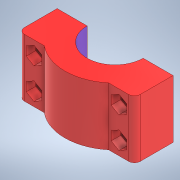
# Autodesk Inventor part: 3_Connettore_inf_INF
Saved by Autodesk Inventor 2020.2 (Build 242310000, 310)
## iProperties
Created: 2019-10-11
Part Number: 3_Connettore_inf_INF
Material: PLA(Stampato)(D0,646)
Document SubType Name: Modeling
Designer: socci
Density: 0.646 g/cm^3
Appearance: Rosso chiaro
Mass: 17.9754 g
Surface Area: 86.3527 cm^2
Volume: 27.8257 cm^3
Author: socci
Autodesk Inventor part; units mm, degrees
ref_plane "YZ Plane" through (0, 0, 0) normal (1, 0, 0) x (0, 1, 0)
ref_plane "XZ Plane" through (0, 0, 0) normal (0, 1, 0) x (-1, 0, 0)
ref_plane "XY Plane" through (0, 0, 0) normal (0, 0, 1) x (1, 0, 0)
sketch "Schizzo1" plane through (0, 0, 0) normal (0, 0, 1) x (1, 0, 0)
  line L0 (-30, -15) -> (30, -15)
  line L1 (30, -15) -> (30, 15)
  line L2 (30, 15) -> (-30, 15)
  line L3 (-30, 15) -> (-30, -15)
  line L4 (-30, -15) -> (30, 15) construction
  line L5 (30, -15) -> (-30, 15) construction
  point P0 (0, 0)
  point P1 (0, 0)
  dimension "d27" = 30
  dimension "d28" = 60
  constraints: 12 end point, 3 midpoint, 2 parallel, 1 horizontal, 1 perpendicular
  measures "d27" distance of L0.end L1.end
  measures "d28" distance of L0.start L0.end
extrude "Estrusione1" add sketch "Schizzo1" against normal blind 20
sketch "Schizzo2" plane through (-25, 15, 0) normal (0, 1, 0) x (1, 0, 0)
  line L0 (55, 20) -> (-5, 20) projected
  circle A0 centre (25, 20) radius 14.5
  point P0 (25, 0)
  dimension "d60" = 29
  dimension "d61" = 20
  constraints: 1 centre point, 1 coincident, 1 midpoint
  measures "d60" diameter of A0
  measures "d61" distance of point (25, 0) A0.centre
extrude "Estrusione2" cut sketch "Schizzo2" against normal blind 30
sketch "Schizzo6" plane through (0, 0, 0) normal (0, 0, 1) x (1, 0, 0)
  line L0 (0, 15) -> (0, 8)
  line L1 (0, 8) -> (-22, 8)
  line L2 (-22, 8) -> (-22, -8)
  line L3 (0, 8) -> (22, 8)
  line L4 (0, 8) -> (22, 8) construction
  line L5 (22, 8) -> (22, -8)
  point P0 (0, 0)
  dimension "d29" = 7
  dimension "d30" = 22
  dimension "d31" = 90
  dimension "d32" = 16
  dimension "d33" = 90
  dimension "d34" = 22
  dimension "d36" = 16
  dimension "d37" = 90
  constraints: 12 end point, 3 perpendicular, 2 horizontal, 1 collinear, 1 vertical
  measures "d29" distance of L0.start L0.end
  measures "d30" distance of L0.end L1.end
  measures "d31" angle of L0 L1
  measures "d32" distance of L1.end L2.end
  measures "d33" angle of L2 L1
  measures "d34" distance of L0.end L3.end
  measures "d36" distance of L3.end L5.end
  measures "d37" angle of L3 L5
hole "Foro3" at (-22, 8, 0) at (-22, -8, 0) at (22, -8, 0) at (22, 8, 0) direction (0, 0, -1) diameter 4.9 end through all clearance for "Vite a testa piana" size "M4" standard "ANSI - Profilo M Metrico"
sketch "Schizzo7" plane through (0, 0, 0) normal (0, 0, 1) x (1, 0, 0)
  line L0 (-14.5, 15) -> (14.5, 15)
  line L1 (0, 15) -> (0, 8)
  line L2 (0, 8) -> (-22, 8)
  line L3 (-22, 8) -> (-22, -8)
  line L4 (0, 8) -> (22, 8)
  line L5 (0, 8) -> (22, 8) construction
  line L6 (22, 8) -> (22, -8)
  circle A0 centre (-22, -8) radius 4
  circle A1 centre (22, 8) radius 4
  circle A2 centre (22, -8) radius 4
  circle A3 centre (-22, 8) radius 4
  line L7 (-18, 5.6906) -> (-22, 3.3812)
  line L8 (-22, 3.3812) -> (-26, 5.6906)
  line L9 (-26, 5.6906) -> (-26, 10.3094)
  line L10 (-26, 10.3094) -> (-22, 12.6188)
  line L11 (-22, 12.6188) -> (-18, 10.3094)
  line L12 (-18, 10.3094) -> (-18, 5.6906)
  line L13 (-18, -10.3094) -> (-22, -12.6188)
  line L14 (-22, -12.6188) -> (-26, -10.3094)
  line L15 (-26, -10.3094) -> (-26, -5.6906)
  line L16 (-26, -5.6906) -> (-22, -3.3812)
  line L17 (-22, -3.3812) -> (-18, -5.6906)
  line L18 (-18, -5.6906) -> (-18, -10.3094)
  line L19 (26, -10.3094) -> (22, -12.6188)
  line L20 (22, -12.6188) -> (18, -10.3094)
  line L21 (18, -10.3094) -> (18, -5.6906)
  line L22 (18, -5.6906) -> (22, -3.3812)
  line L23 (22, -3.3812) -> (26, -5.6906)
  line L24 (26, -5.6906) -> (26, -10.3094)
  line L25 (26, 5.6906) -> (22, 3.3812)
  line L26 (22, 3.3812) -> (18, 5.6906)
  line L27 (18, 5.6906) -> (18, 10.3094)
  line L28 (18, 10.3094) -> (22, 12.6188)
  line L29 (22, 12.6188) -> (26, 10.3094)
  line L30 (26, 10.3094) -> (26, 5.6906)
  point P0 (0, 0)
  point P1 (0, 0)
  point P2 (-18, 8)
  point P3 (-18, -8)
  point P4 (26, -8)
  point P5 (26, 8)
  point P6 (-24, -11.4641)
  point P7 (-20, -11.4641)
  point P8 (-26, -8)
  point P9 (-24, -4.5359)
  point P10 (-20, -4.5359)
  dimension "d54" = 8
  dimension "d55" = 8
  dimension "d56" = 8
  dimension "d69" = 8
  dimension "d45" = 7
  dimension "d46" = 22
  dimension "d47" = 90
  dimension "d48" = 16
  dimension "d49" = 90
  dimension "d50" = 22
  dimension "d51" = 16
  constraints: 62 end point, 7 coincident, 5 midpoint, 3 horizontal alignment, 3 perpendicular, 2 horizontal, 1 collinear, 1 point on line, 1 vertical, 61 other
  measures "d45" distance of L1.start L1.end
  measures "d46" distance of L1.end L2.end
  measures "d47" angle of L1 L2
  measures "d48" distance of L2.end L3.end
  measures "d49" angle of L3 L2
  measures "d50" distance of L1.end L4.end
  measures "d51" distance of L4.end L6.end
extrude "Estrusione4" cut sketch "Schizzo7" against normal blind 5
fillet "Raccordo1" radius 3 1 edges at (30, 0, 0)
fillet "Raccordo2" radius 3 1 edges at (-30, 0, 0)
sketch "Schizzo9" plane through (0, 15, -20) normal (0, 1, 0) x (1, 0, 0)
  circle A0 centre (0, 0) radius 26
  line L0 (27, -20) -> (-27, -20) projected
  line L1 (16.6132, -20) -> (-16.6132, -20)
  point P0 (0, -20)
  dimension "d66" = 52
  constraints: 2 end point, 2 point on circle, 2 point on line, 1 centre point
  measures "d66" diameter of A0
extrude "Estrusione5" add sketch "Schizzo9" against normal blind 30 contours L0 A0 picked at (-3.8639, -21.091)
